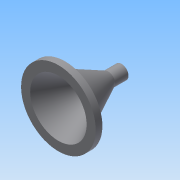
# Autodesk Inventor part: nozzletopcone
Saved by Autodesk Inventor 2015 SP1 (Build 190203100, 203)
## iProperties
Created: 2015-04-28
Part Number: nozzletopcone
Material: Generic
Document SubType Name: Modeling
Designer: Admin
Density: 1 g/cm^3
Appearance: Default
Author: Admin
Autodesk Inventor part; units mm, degrees
ref_plane "YZ Plane" through (0, 0, 0) normal (1, 0, 0) x (0, 1, 0)
ref_plane "XZ Plane" through (0, 0, 0) normal (0, 1, 0) x (-1, 0, 0)
ref_plane "XY Plane" through (0, 0, 0) normal (0, 0, 1) x (1, 0, 0)
sketch "Sketch1" plane through (0, 0, 0) normal (1, 0, 0) x (0, 1, 0)
  line L0 (0, 17.78) -> (3.175, 17.78)
  line L1 (3.175, 17.78) -> (3.175, 13.462)
  line L2 (0, 0) -> (30.099, 0)
  line L3 (30.099, 0) -> (30.099, 3.2908)
  line L4 (30.099, 3.2908) -> (23.7557, 3.2908)
  line L5 (23.7557, 3.2908) -> (3.175, 13.462)
  line L6 (23.7557, 0) -> (0, 13.462)
  line L7 (0, 17.78) -> (0, 13.462)
  dimension "d0" = 17.78
  dimension "d1" = 3.175
  dimension "d2" = 4.318
  dimension "d3" = 30.099
  constraints: 16 end point, 3 vertical, 2 horizontal, 1 perpendicular, 1 point on line
  measures "d0" distance of L2.start L0.start
  measures "d1" distance of L0.start L0.end
  measures "d2" distance of L0.end L1.end
  measures "d3" distance of L2.start L2.end
revolve "Revolution1" add sketch "Sketch1" angle 360 about axis through (0, 0, 0) along (0, 1, 0)
body "Solid1"
